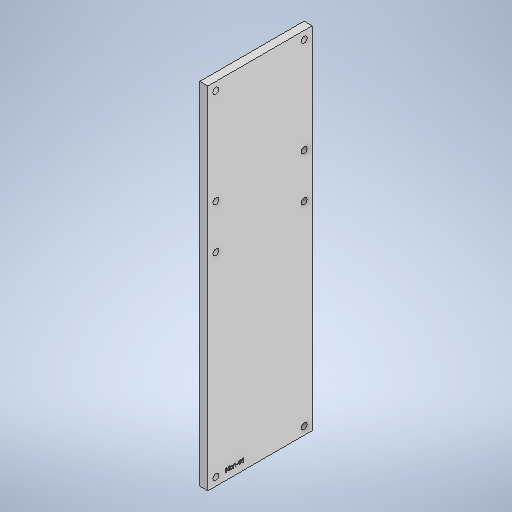
# Autodesk Inventor part: Tilt Slide
Saved by Autodesk Inventor 2025 (Build 290162000, 162)
## iProperties
Created: 2024-10-25
Part Number: Tilt Slide
Material: Generic
Document SubType Name: Modeling
Designer: liaco
Density: 1 g/cm^3
Appearance: Default
Mass: 103.146 g
Surface Area: 522.762 cm^2
Volume: 103.146 cm^3
Author: liaco
Autodesk Inventor part; units mm, degrees
ref_plane "YZ Plane" through (0, 0, 0) normal (1, 0, 0) x (0, 1, 0)
ref_plane "XZ Plane" through (0, 0, 0) normal (0, 1, 0) x (-1, 0, 0)
ref_plane "XY Plane" through (0, 0, 0) normal (0, 0, 1) x (1, 0, 0)
sketch "Sketch1" plane through (0, 0, 0) normal (1, 0, 0) x (0, 1, 0)
  line L0 (262, 78) -> (0, 78)
  line L1 (0, 78) -> (0, 0)
  line L2 (0, 0) -> (262, 0)
  line L3 (262, 0) -> (262, 78)
  point P0 (0, 0)
  point P1 (131, 0)
  dimension "d0" = 262
  dimension "d1" = 78
  dimension "d2" = 0
  dimension "d3" = 0
  constraints: 8 end point, 2 parallel, 1 horizontal, 1 midpoint, 1 perpendicular
  measures "d0" distance of L1.end L2.end
  measures "d1" distance of L2.end L0.start
  measures "d2" vertical distance of point (131, 0) point (0, 0)
  measures "d3" distance from line of L1 point (0, 0)
extrude "Extrusion1" add sketch "Sketch1" along normal blind 6
sketch "Sketch13" plane through (6, 0, 0) normal (1, 0, 0) x (0, 0, -1)
  line L0 (-78, 262) -> (-78, 0) projected
  line L1 (0, 262) -> (-78, 262) projected
  line L2 (0, 0) -> (0, 262) projected
  line L3 (-78, 0) -> (0, 0) projected
  line L4 (-78, 168) -> (0, 168)
  line L5 (-77, 172.5) -> (-1, 163.5) construction
  line L6 (-1, 172.5) -> (-77, 163.5) construction
  point P0 (-72, 256)
  point P1 (-6, 256)
  point P2 (-72, 6)
  point P3 (-6, 6)
  point P4 (-39, 168)
  point P5 (-6, 151.5)
  point P6 (-72, 151.5)
  point P7 (-6, 184.5)
  point P8 (-72, 184.5)
  dimension "d124" = 6
  dimension "d125" = 6
  dimension "d126" = 6
  dimension "d127" = 6
  dimension "d128" = 6
  dimension "d129" = 6
  dimension "d130" = 6
  dimension "d131" = 6
  dimension "d132" = 88
  dimension "d134" = 6
  dimension "d135" = 6
  dimension "d145" = 16.5
  dimension "d146" = 16.5
  constraints: 6 end point, 3 midpoint, 2 point on line, 2 symmetric about line, 1 perpendicular
  measures "d124" distance from line of point (-72, 256) L0
  measures "d125" distance from line of L1 point (-72, 256)
  measures "d126" distance from line of L1 point (-6, 256)
  measures "d127" distance from line of L2 point (-6, 256)
  measures "d128" distance from line of L3 point (-72, 6)
  measures "d129" distance from line of L0 point (-72, 6)
  measures "d130" distance from line of L2 point (-6, 6)
  measures "d131" distance from line of L3 point (-6, 6)
  measures "d132" distance from line of L4 point (-72, 256)
  measures "d134" distance from line of L2 point (-6, 151.5)
  measures "d135" distance from line of L0 point (-72, 151.5)
  measures "d145" distance from line of L4 point (-6, 151.5)
  measures "d146" distance from line of L4 point (-72, 151.5)
hole "Hole5" at (6, 256, 72) at (6, 256, 6) at (6, 6, 72) at (6, 6, 6) at (6, 151.5, 6) at (6, 151.5, 72) at (6, 184.5, 72) at (6, 184.5, 6) direction (-1, 0, 0) diameter 4.5 end through all clearance for "Flat Head Machine Screw" size "M4" standard "Ansi Metric M Profile"
sketch "Sketch14" plane through (6, 0, 0) normal (1, 0, 0) x (0, 0, -1)
  line L0 (-64.8549, 8.2591) -> (-35.082, 8.2591) construction
  line L1 (-35.082, 8.2591) -> (-35.082, -0.7555) construction
  line L2 (-35.082, -0.7555) -> (-64.8549, -0.7555) construction
  line L3 (-64.8549, -0.7555) -> (-64.8549, 8.2591) construction
  line L4 (-61.9329, 5.1543) -> (-62.338, 5.1543)
  line L5 (-62.338, 5.1543) -> (-62.338, 7.7799)
  line L6 (-62.338, 7.7799) -> (-63.1333, 5.9941)
  line L7 (-63.1333, 5.9941) -> (-63.3803, 5.9941)
  line L8 (-63.3803, 5.9941) -> (-64.1683, 7.7799)
  line L9 (-64.1683, 7.7799) -> (-64.1683, 5.1543)
  line L10 (-64.1683, 5.1543) -> (-64.5462, 5.1543)
  line L11 (-64.5462, 5.1543) -> (-64.5462, 8.2023)
  line L12 (-64.5462, 8.2023) -> (-63.9929, 8.2023)
  line L13 (-63.9929, 8.2023) -> (-63.2321, 6.5054)
  line L14 (-63.2321, 6.5054) -> (-62.4961, 8.2023)
  line L15 (-62.4961, 8.2023) -> (-61.9329, 8.2023)
  line L16 (-61.9329, 8.2023) -> (-61.9329, 5.1543)
  spline S0 degree 2 poles (-59.4654, 6.2979) (-59.4654, 5.7199) (-60.0211, 5.0901) (-60.4855, 5.0901) knots 0 0 0 1 2 2 2
  spline S1 degree 2 poles (-60.4855, 5.0901) (-60.9622, 5.0901) (-61.5081, 5.7397) (-61.5081, 6.2979) knots 0 0 0 1 2 2 2
  spline S2 degree 2 poles (-61.5081, 6.2979) (-61.5081, 6.8709) (-60.9449, 7.5057) (-60.4855, 7.5057) knots 0 0 0 1 2 2 2
  spline S3 degree 2 poles (-60.4855, 7.5057) (-60.0211, 7.5057) (-59.4654, 6.8734) (-59.4654, 6.2979) knots 0 0 0 1 2 2 2
  spline S4 degree 2 poles (-59.863, 6.2979) (-59.863, 6.7425) (-60.1866, 7.1748) (-60.4855, 7.1748) knots 0 0 0 1 2 2 2
  spline S5 degree 2 poles (-60.4855, 7.1748) (-60.7843, 7.1748) (-61.1104, 6.7425) (-61.1104, 6.2979) knots 0 0 0 1 2 2 2
  spline S6 degree 2 poles (-61.1104, 6.2979) (-61.1104, 5.8656) (-60.7843, 5.421) (-60.4855, 5.421) knots 0 0 0 1 2 2 2
  spline S7 degree 2 poles (-60.4855, 5.421) (-60.1891, 5.421) (-59.863, 5.8582) (-59.863, 6.2979) knots 0 0 0 1 2 2 2
  line L17 (-57.2744, 5.1543) -> (-57.6598, 5.1543)
  line L18 (-57.6598, 5.1543) -> (-57.6598, 6.4584)
  spline S8 degree 2 poles (-57.6598, 6.4584) (-57.6598, 6.6165) (-57.6894, 6.8882) (-57.7339, 6.9697) knots 0 0 0 1 2 2 2
  spline S9 degree 2 poles (-57.7339, 6.9697) (-57.7808, 7.0562) (-57.9488, 7.1402) (-58.092, 7.1402) knots 0 0 0 1 2 2 2
  spline S10 degree 2 poles (-58.092, 7.1402) (-58.2353, 7.1402) (-58.5391, 6.987) (-58.6848, 6.8635) knots 0 0 0 1 2 2 2
  line L19 (-58.6848, 6.8635) -> (-58.6848, 5.1543)
  line L20 (-58.6848, 5.1543) -> (-59.0702, 5.1543)
  line L21 (-59.0702, 5.1543) -> (-59.0702, 7.4415)
  line L22 (-59.0702, 7.4415) -> (-58.6848, 7.4415)
  line L23 (-58.6848, 7.4415) -> (-58.6848, 7.1871)
  spline S11 degree 2 poles (-58.6848, 7.1871) (-58.5119, 7.3427) (-58.1785, 7.5057) (-57.9908, 7.5057) knots 0 0 0 1 2 2 2
  spline S12 degree 2 poles (-57.9908, 7.5057) (-57.6548, 7.5057) (-57.2744, 7.0611) (-57.2744, 6.6388) knots 0 0 0 1 2 2 2
  line L24 (-57.2744, 6.6388) -> (-57.2744, 5.1543)
  line L25 (-55.6739, 6.3028) -> (-56.8274, 6.3028)
  line L26 (-56.8274, 6.3028) -> (-56.8274, 6.6733)
  line L27 (-56.8274, 6.6733) -> (-55.6739, 6.6733)
  line L28 (-55.6739, 6.6733) -> (-55.6739, 6.3028)
  line L29 (-53.3076, 6.2016) -> (-53.6707, 6.2016)
  line L30 (-53.6707, 6.2016) -> (-53.6707, 5.1543)
  line L31 (-53.6707, 5.1543) -> (-54.0634, 5.1543)
  line L32 (-54.0634, 5.1543) -> (-54.0634, 6.2016)
  line L33 (-54.0634, 6.2016) -> (-55.4096, 6.2016)
  line L34 (-55.4096, 6.2016) -> (-55.4096, 6.6313)
  line L35 (-55.4096, 6.6313) -> (-54.0461, 8.2023)
  line L36 (-54.0461, 8.2023) -> (-53.6707, 8.2023)
  line L37 (-53.6707, 8.2023) -> (-53.6707, 6.5301)
  line L38 (-53.6707, 6.5301) -> (-53.3076, 6.5301)
  line L39 (-53.3076, 6.5301) -> (-53.3076, 6.2016)
  line L40 (-54.0634, 6.5301) -> (-54.0634, 7.7206)
  line L41 (-54.0634, 7.7206) -> (-55.0885, 6.5301)
  line L42 (-55.0885, 6.5301) -> (-54.0634, 6.5301)
  spline S13 degree 2 poles (-51.0549, 6.1423) (-51.0549, 5.9076) (-51.2106, 5.51) (-51.3415, 5.3766) knots 0 0 0 1 2 2 2
  spline S14 degree 2 poles (-51.3415, 5.3766) (-51.4773, 5.2358) (-51.8182, 5.0901) (-52.0232, 5.0901) knots 0 0 0 1 2 2 2
  spline S15 degree 2 poles (-52.0232, 5.0901) (-52.2282, 5.0901) (-52.5666, 5.2284) (-52.695, 5.3667) knots 0 0 0 1 2 2 2
  spline S16 degree 2 poles (-52.695, 5.3667) (-52.8531, 5.5322) (-53.031, 6.0879) (-53.031, 6.493) knots 0 0 0 1 2 2 2
  spline S17 degree 2 poles (-53.031, 6.493) (-53.031, 6.8907) (-52.8679, 7.5304) (-52.6975, 7.7676) knots 0 0 0 1 2 2 2
  spline S18 degree 2 poles (-52.6975, 7.7676) (-52.532, 7.9997) (-52.0084, 8.2591) (-51.665, 8.2591) knots 0 0 0 1 2 2 2
  spline S19 degree 2 poles (-51.665, 8.2591) (-51.5638, 8.2591) (-51.3859, 8.2393) (-51.3192, 8.2171) knots 0 0 0 1 2 2 2
  line L43 (-51.3192, 8.2171) -> (-51.3192, 7.8244)
  line L44 (-51.3192, 7.8244) -> (-51.3365, 7.8244)
  spline S20 degree 2 poles (-51.3365, 7.8244) (-51.3933, 7.854) (-51.6008, 7.9059) (-51.7194, 7.9059) knots 0 0 0 1 2 2 2
  spline S21 degree 2 poles (-51.7194, 7.9059) (-52.0998, 7.9059) (-52.5666, 7.3921) (-52.6111, 6.8882) knots 0 0 0 1 2 2 2
  spline S22 degree 2 poles (-52.6111, 6.8882) (-52.4653, 6.9895) (-52.159, 7.1007) (-51.9763, 7.1007) knots 0 0 0 1 2 2 2
  spline S23 degree 2 poles (-51.9763, 7.1007) (-51.7984, 7.1007) (-51.5317, 7.029) (-51.3859, 6.9203) knots 0 0 0 1 2 2 2
  spline S24 degree 2 poles (-51.3859, 6.9203) (-51.218, 6.7944) (-51.0549, 6.4041) (-51.0549, 6.1423) knots 0 0 0 1 2 2 2
  spline S25 degree 2 poles (-51.4699, 6.125) (-51.4699, 6.3127) (-51.5687, 6.5671) (-51.6774, 6.656) knots 0 0 0 1 2 2 2
  spline S26 degree 2 poles (-51.6774, 6.656) (-51.7589, 6.7203) (-51.9614, 6.7623) (-52.0677, 6.7623) knots 0 0 0 1 2 2 2
  spline S27 degree 2 poles (-52.0677, 6.7623) (-52.2109, 6.7623) (-52.4801, 6.6758) (-52.6111, 6.5943) knots 0 0 0 1 2 2 2
  spline S28 degree 2 poles (-52.6111, 6.5943) (-52.6135, 6.5498) (-52.6185, 6.4659) (-52.6185, 6.4016) knots 0 0 0 1 2 2 2
  spline S29 degree 2 poles (-52.6185, 6.4016) (-52.6185, 6.0855) (-52.495, 5.6977) (-52.4011, 5.5964) knots 0 0 0 1 2 2 2
  spline S30 degree 2 poles (-52.4011, 5.5964) (-52.3147, 5.5001) (-52.1269, 5.4235) (-52.0207, 5.4235) knots 0 0 0 1 2 2 2
  spline S31 degree 2 poles (-52.0207, 5.4235) (-51.7737, 5.4235) (-51.4699, 5.7743) (-51.4699, 6.125) knots 0 0 0 1 2 2 2
  point P0 (0, 0)
  constraints: 2 other
extrude "Extrusion8" cut sketch "Sketch14" against normal blind 0.5
body "Solid1"
